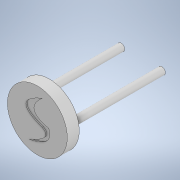
# Autodesk Inventor part: Photoresistor
Saved by Autodesk Inventor 2021 (Build 250183000, 183)
## iProperties
Created: 2021-07-28
Part Number: Photoresistor
Material: Generic
Document SubType Name: Modeling
Designer: USER
Density: 1 g/cm^3
Appearance: Default
Author: USER
Autodesk Inventor part; units mm, degrees
ref_plane "YZ Plane" through (0, 0, 0) normal (1, 0, 0) x (0, 1, 0)
ref_plane "XZ Plane" through (0, 0, 0) normal (0, 1, 0) x (-1, 0, 0)
ref_plane "XY Plane" through (0, 0, 0) normal (0, 0, 1) x (1, 0, 0)
sketch "Sketch1" plane through (0, 0, 0) normal (0, 0, 1) x (1, 0, 0)
  circle A0 centre (0, 0) radius 25
  line L0 (9.0545, 19) -> (-15.9277, 6.5172) construction
  line L1 (-15.9277, 6.5172) -> (4.4593, -0.1187) construction
  line L2 (4.4593, -0.1187) -> (8.9648, -0.1187) construction
  line L3 (8.9648, -0.1187) -> (-5.7342, -19.5656) construction
  line L4 (-5.7342, -19.5656) -> (-5.7342, -19.5656) construction
  spline S0 degree 4 poles (9.0545, 19) (-15.9277, 6.5172) (4.4593, -0.1187) (8.9648, -0.1187) (-5.7195, -19.5462) (-5.7342, -19.5656) knots 1 1 1 1 1 2 3 3 3 3 3
  line L5 (9.0545, 19) -> (1.8467, 5.2615) construction
  line L6 (1.8467, 5.2615) -> (8.9648, -0.1187) construction
  line L7 (8.9648, -0.1187) -> (9.0545, 0) construction
  line L8 (9.0545, 0) -> (4.4598, -12) construction
  line L9 (4.4598, -12) -> (-5.7342, -19.5656) construction
  spline S1 degree 4 poles (9.0545, 19) (1.8467, 5.2615) (8.9648, -0.1187) (9.0545, 0) (4.4598, -12) (-5.7342, -19.5656) knots 1 1 1 1 1 2 3 3 3 3 3
  constraints: 3 coincident, 2 horizontal, 1 centre point, 1 point on line, 6 other
extrude "Extrusion1" add sketch "Sketch1" against normal blind 10 contours A0 | S1 S0
sketch "Sketch2" plane through (0, 0, 0) normal (0, 0, 1) x (1, 0, 0)
  line L0 (4, 18) -> (-23, 7) construction
  line L1 (-23, 7) -> (4, -3) construction
  spline S0 degree 2 poles (4, 18) (-23, 7) (4, -3) knots 1 1 1 2 2 2
  line L2 (4, -3) -> (15.0435, -8.5217) construction
  line L3 (15.0435, -8.5217) -> (-7, -17) construction
  line L4 (-7, -17) -> (-7.0477, -17) construction
  spline S1 degree 3 poles (4, -3) (15.0435, -8.5217) (-7, -17) (-7.0477, -17) knots 1 1 1 1 2 2 2 2
  line L5 (4, 18) -> (-12, 4) construction
  line L6 (-12, 4) -> (9.5217, -1) construction
  spline S2 degree 2 poles (4, 18) (-12, 4) (9.5217, -1) knots 1 1 1 2 2 2
  line L7 (9.5217, -1) -> (14.1934, -13.1463) construction
  line L8 (14.1934, -13.1463) -> (-7.0477, -17) construction
  spline S3 degree 2 poles (9.5217, -1) (14.1934, -13.1463) (-7.0477, -17) knots 1 1 1 2 2 2
  point P0 (0, 0)
  constraints: 1 horizontal, 1 perpendicular, 12 other
extrude "Extrusion2" cut sketch "Sketch2" against normal blind 0.9
sketch "Sketch3" plane through (0, 0, -10) normal (0, 0, -1) x (-1, 0, 0)
  circle A0 centre (-16, 0) radius 3
  circle A1 centre (18, 0) radius 3
  point P0 (0, 0)
  constraints: 2 centre point
extrude "Extrusion3" add sketch "Sketch3" along normal blind 78
body "Solid1"
